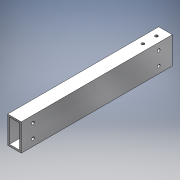
# Autodesk Inventor part: オムニ_角柱6
Saved by Autodesk Inventor 2019.4 (Build 234330000, 330)
## iProperties
Created: 2021-12-04
Part Number: オムニ_角柱6
Material: アルミニウム 6061
Document SubType Name: Modeling
Designer: 堀川皓史
Density: 2.7 g/cm^3
Appearance: アルミニウム - フラット
Author: 堀川皓史
Autodesk Inventor part; units mm, degrees
ref_plane "YZ Plane" through (0, 0, 0) normal (1, 0, 0) x (0, 1, 0)
ref_plane "XZ Plane" through (0, 0, 0) normal (0, 1, 0) x (-1, 0, 0)
ref_plane "XY Plane" through (0, 0, 0) normal (0, 0, 1) x (1, 0, 0)
sketch "スケッチ1" plane through (0, 0, 0) normal (0, 0, 1) x (1, 0, 0)
  line L0 (7.5, 15) -> (-7.5, 15)
  line L1 (-7.5, 15) -> (-7.5, -15)
  line L2 (-7.5, -15) -> (7.5, -15)
  line L3 (7.5, -15) -> (7.5, 15)
  line L4 (7.5, 15) -> (-7.5, -15) construction
  line L5 (-7.5, 15) -> (7.5, -15) construction
  line L6 (-5.5, 13) -> (5.5, 13)
  line L7 (5.5, 13) -> (5.5, -13)
  line L8 (5.5, -13) -> (-5.5, -13)
  line L9 (-5.5, -13) -> (-5.5, 13)
  point P0 (0, 0)
  dimension "d2" = 15
  dimension "d3" = 30
  dimension "d4" = 2
  constraints: 20 end point, 4 parallel, 2 midpoint, 2 perpendicular, 1 horizontal, 3 other
  measures "d2" distance of L2.end L1.end
  measures "d3" distance of L1.end L0.end
  measures "d4" distance between parallel lines of L0 L6
extrude "押し出し1" add sketch "スケッチ1" along normal blind 167
sketch "スケッチ2" plane through (7.5, -15, 0) normal (1, 0, 0) x (0, 0, -1)
  circle A0 centre (-15, 22.5) radius 1.6
  circle A1 centre (-15, 7.5) radius 1.6
  circle A2 centre (-154, 22.5) radius 1.6
  circle A3 centre (-154, 7.5) radius 1.6
  line L0 (0, 30) -> (-167, 30) projected
  point P0 (0, 15)
  dimension "d7" = 3.2
  dimension "d8" = 3.2
  dimension "d9" = 3.2
  dimension "d10" = 3.2
  dimension "d11" = 15
  dimension "d12" = 15
  dimension "d13" = 7.5
  dimension "d14" = 139
  constraints: 4 centre point, 2 horizontal alignment, 2 vertical alignment
  measures "d7" diameter of A0
  measures "d8" diameter of A1
  measures "d9" diameter of A2
  measures "d10" diameter of A3
  measures "d11" horizontal distance of point (0, 15) A0.centre
  measures "d12" distance of A1.centre A0.centre
  measures "d13" distance from line of L0 A0.centre
  measures "d14" distance of A1.centre A3.centre
extrude "押し出し2" cut sketch "スケッチ2" against normal through all
sketch "スケッチ4" plane through (-7.5, 15, 0) normal (0, 1, 0) x (1, 0, 0)
  circle A0 centre (7.5, -10) radius 1.6
  circle A1 centre (7.5, -25) radius 1.6
  line L0 (15, 0) -> (0, 0) projected
  point P0 (7.5, 0)
  point P1 (7.5, 0)
  dimension "d17" = 3.2
  dimension "d18" = 3.2
  dimension "d19" = 15
  dimension "d20" = 10
  constraints: 2 centre point, 2 vertical alignment, 1 midpoint
  measures "d17" diameter of A0
  measures "d18" diameter of A1
  measures "d19" distance of A1.centre A0.centre
  measures "d20" distance of point (7.5, 0) A0.centre
extrude "押し出し3" cut sketch "スケッチ4" against normal through all
